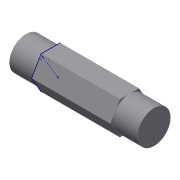
# Autodesk Inventor part: LongShaft
Saved by Autodesk Inventor 2013 SP1 (Build 170176100, 176)
## iProperties
Created: 2013-11-18
Part Number: LongShaft
Material: Generic
Document SubType Name: Modeling
Designer: robotics
Density: 1 g/cm^3
Author: robotics
Autodesk Inventor part; units mm, degrees
ref_plane "YZ Plane" through (0, 0, 0) normal (1, 0, 0) x (0, 1, 0)
ref_plane "XZ Plane" through (0, 0, 0) normal (0, 1, 0) x (-1, 0, 0)
ref_plane "XY Plane" through (0, 0, 0) normal (0, 0, 1) x (1, 0, 0)
sketch "Sketch1" plane through (0, 0, 0) normal (1, 0, 0) x (0, 1, 0)
  line L0 (5.4993, 0) -> (2.7496, -4.7625)
  line L1 (2.7496, -4.7625) -> (-2.7496, -4.7625)
  line L2 (-2.7496, -4.7625) -> (-5.4993, 0)
  line L3 (-5.4993, 0) -> (-2.7496, 4.7625)
  line L4 (-2.7496, 4.7625) -> (2.7496, 4.7625)
  line L5 (2.7496, 4.7625) -> (5.4993, 0)
  circle A0 centre (0, 0) radius 4.7625
  dimension "d0" = 9.525
  constraints: 12 end point, 2 coincident, 1 centre point, 1 horizontal alignment, 1 tangent, 13 other
  measures "d0" diameter of A0
extrude "Extrusion1" add sketch "Sketch1" along normal blind 26.2984
extrude "Extrusion2" add sketch "Sketch1" against normal blind 7.112 contours A0
sketch "Sketch3" plane through (26.2984, 0, 0) normal (1, 0, 0) x (0, 0, -1)
  line L0 (0, 5.4993) -> (-4.7625, 2.7496) projected
  circle A0 centre (0, 0) radius 4.7625
  constraints: 1 centre point, 1 coincident, 1 tangent
extrude "Extrusion3" add sketch "Sketch3" along normal blind 7.112
body "Solid1"
